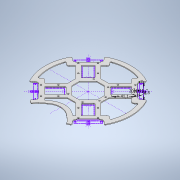
# Autodesk Inventor part: wooden_plate
Saved by Autodesk Inventor 2020 (Build 240168000, 168)
## iProperties
Created: 2023-11-06
Part Number: wooden_plate
Material: Типовые
Document SubType Name: Modeling
Designer: denis
Density: 1 g/cm^3
Appearance: По умолчанию
Author: denis
Autodesk Inventor part; units mm, degrees
ref_plane "YZ Plane" through (0, 0, 0) normal (1, 0, 0) x (0, 1, 0)
ref_plane "XZ Plane" through (0, 0, 0) normal (0, 1, 0) x (-1, 0, 0)
ref_plane "XY Plane" through (0, 0, 0) normal (0, 0, 1) x (1, 0, 0)
sketch "Эскиз1" plane through (0, 0, 0) normal (0, 1, 0) x (-1, 0, 0)
  line L0 (36.7845, -19.8139) -> (61.5324, -44.5618)
  line L1 (36.7845, -5.6718) -> (68.6034, -37.4907)
  line L2 (37.4907, -68.6034) -> (5.6718, -36.7845)
  line L3 (0, 0) -> (60.1181, -60.1181) construction
  line L4 (19.8139, -36.7845) -> (44.5618, -61.5324)
  line L5 (32.2885, -89.3342) -> (30.5289, -89.9833)
  arc A0 (-49.5952, -92.5729) -> (48.7112, -93.0411) centre (0, 0) ccw
  arc A1 (-33.5718, -88.8929) -> (30.5289, -89.9833) centre (0, 0) ccw
  arc A2 (36.7845, -19.8139) -> (33.956, -19.8139) centre (35.3703, -21.2281) ccw
  arc A3 (19.8139, -33.956) -> (19.8139, -36.7845) centre (21.2281, -35.3703) ccw
  line L6 (33.956, -19.8139) -> (19.8139, -33.956)
  arc A4 (48.717, 93.0381) -> (45.4357, 94.6838) centre (0, 0) ccw
  line L7 (0, 0) -> (0, 95.3237) construction
  arc A5 (89.9833, 30.5289) -> (-89.9833, 30.5289) centre (0, 0) ccw construction
  line L8 (0, 0) -> (74.2611, 74.2611) construction
  arc A6 (73.9076, 46.3304) -> (85.2213, 46.3304) centre (79.5644, 51.9873) ccw
  line L9 (85.2213, 46.3304) -> (87.5799, 48.689)
  line L10 (-52.2189, 91.1187) -> (-48.7112, 93.0411) construction
  spline S0 degree 2 poles (-48.6736, 87.5645) (-52.2189, 91.1187) (-48.7112, 93.0411) knots 1 1 1 2 2 2
  line L11 (-48.6736, 87.5645) -> (-52.2189, 91.1187) construction
  arc A7 (-46.3155, 73.8927) -> (-46.3155, 85.2064) centre (-51.9723, 79.5495) ccw
  line L12 (-48.6736, 87.5645) -> (-46.3155, 85.2064)
  arc A8 (-45.4357, 94.6838) -> (-48.7112, 93.0411) centre (0, 0) ccw
  line L13 (-46.3155, 73.8927) -> (-73.8927, 46.3155)
  arc A9 (-85.2064, 46.3155) -> (-73.8927, 46.3155) centre (-79.5495, 51.9723) ccw
  line L14 (-85.2064, 46.3155) -> (-87.5645, 48.6736)
  spline S1 degree 2 poles (-87.5645, 48.6736) (-91.1186, 52.2191) (-92.5729, 49.5952) knots 1 1 1 2 2 2
  line L15 (-87.5645, 48.6736) -> (-91.1186, 52.2191) construction
  line L16 (-91.1186, 52.2191) -> (-92.5729, 49.5952) construction
  arc A10 (44.0429, 95.3397) -> (43.5857, 95.5495) centre (0, 0) ccw construction
  arc A11 (46.3304, 85.2213) -> (46.3304, 73.9076) centre (51.9873, 79.5644) ccw
  line L17 (48.689, 87.5799) -> (46.3304, 85.2213)
  spline S2 degree 2 poles (48.689, 87.5799) (52.2246, 91.1154) (48.717, 93.0381) knots 1 1 1 2 2 2
  line L18 (48.689, 87.5799) -> (52.2246, 91.1154) construction
  line L19 (52.2246, 91.1154) -> (48.717, 93.0381) construction
  line L20 (52.2246, 91.1154) -> (48.689, 87.5799) construction
  line L21 (52.2246, 91.1154) -> (48.689, 87.5799) construction
  line L22 (46.3304, 73.9076) -> (73.9076, 46.3304)
  line L23 (91.1154, 52.2246) -> (87.5799, 48.689) construction
  line L24 (91.1154, 52.2246) -> (92.5699, 49.6008) construction
  spline S3 degree 2 poles (87.5799, 48.689) (91.1154, 52.2246) (92.5699, 49.6008) knots 1 1 1 2 2 2
  line L25 (87.5799, 48.689) -> (91.1154, 52.2246) construction
  arc A12 (-92.5729, 49.5952) -> (-92.5729, -49.5952) centre (0, 0) ccw
  arc A13 (-89.9833, 30.5289) -> (-89.9833, -30.5289) centre (0, 0) ccw
  arc A14 (85.2064, -46.3155) -> (73.9068, -46.3295) centre (79.5636, -51.9864) ccw
  line L26 (85.2064, -46.3155) -> (87.5645, -48.6736)
  arc A15 (92.5729, -49.5952) -> (92.5699, 49.6008) centre (0, 0) ccw
  line L27 (-86.0436, 33.0106) -> (-83.1, 30.067)
  arc A16 (-86.0436, 33.0106) -> (-89.3342, 32.2885) centre (-87.4578, 31.5964) ccw
  line L28 (-89.3342, 32.2885) -> (-89.9833, 30.5289)
  line L29 (91.1154, 52.2246) -> (92.5699, 49.6008) construction
  line L30 (-76.0289, 30.067) -> (-35.2838, 70.8121)
  line L31 (76.0289, 30.067) -> (33.524, 72.5718)
  arc A17 (-48.7112, 93.0411) -> (-92.5729, 49.5952) centre (0, 0) ccw construction
  line L32 (52.2246, 91.1154) -> (48.717, 93.0381) construction
  line L33 (87.5799, 48.689) -> (91.1154, 52.2246) construction
  arc A18 (92.5699, 49.6008) -> (48.717, 93.0381) centre (0, 0) ccw construction
  line L34 (91.1154, 52.2246) -> (52.2246, 91.1154) construction
  line L35 (86.0436, 33.0106) -> (83.1, 30.067)
  arc A19 (89.3342, 32.2885) -> (86.0436, 33.0106) centre (87.4578, 31.5964) ccw
  line L36 (89.3342, 32.2885) -> (89.9833, 30.5289)
  arc A20 (83.7601, -44.8693) -> (89.9833, -30.5289) centre (0, 0) ccw construction
  line L37 (86.0436, -33.0106) -> (83.0991, -30.0661)
  line L38 (89.3342, -32.2885) -> (89.9833, -30.5289)
  arc A21 (86.0436, -33.0106) -> (89.3342, -32.2885) centre (87.4578, -31.5964) ccw
  arc A22 (89.9833, -30.5289) -> (89.9833, 30.5289) centre (0, 0) ccw
  arc A23 (83.0991, -30.0661) -> (76.0281, -30.0661) centre (79.5636, -33.6016) ccw
  arc A24 (30.0661, -76.0281) -> (30.0661, -83.0991) centre (33.6016, -79.5636) ccw
  line L39 (33.0106, -86.0436) -> (30.0661, -83.0991)
  spline S4 degree 2 poles (48.6736, -87.5645) (52.2189, -91.1187) (48.7112, -93.0411) knots 1 1 1 2 2 2
  line L40 (48.6736, -87.5645) -> (52.2189, -91.1187) construction
  line L41 (52.2189, -91.1187) -> (48.7112, -93.0411) construction
  arc A25 (32.2885, -89.3342) -> (33.0106, -86.0436) centre (31.5964, -87.4578) ccw
  line L42 (48.6736, -87.5645) -> (46.3147, -85.2055)
  line L43 (48.6736, -87.5645) -> (46.3147, -85.2055) construction
  arc A26 (46.3295, -73.9068) -> (46.3147, -85.2055) centre (51.9864, -79.5636) ccw
  line L44 (76.0281, -30.0661) -> (30.0661, -76.0281)
  line L45 (46.3295, -73.9068) -> (73.9068, -46.3295)
  line L46 (46.3295, -73.9068) -> (73.9068, -46.3295) construction
  line L47 (73.9068, -46.3295) -> (46.3295, -73.9068) construction
  arc A27 (30.5289, -89.9833) -> (83.7601, -44.8693) centre (0, 0) ccw construction
  line L48 (87.5645, -48.6736) -> (91.1186, -52.2191) construction
  spline S5 degree 2 poles (87.5645, -48.6736) (91.1186, -52.2191) (92.5729, -49.5952) knots 1 1 1 2 2 2
  line L49 (91.1186, -52.2191) -> (92.5729, -49.5952) construction
  arc A28 (48.7112, -93.0411) -> (92.5729, -49.5952) centre (0, 0) ccw construction
  line L50 (0, 51.9187) -> (0, 56.4187) construction
  arc A29 (76.0289, 30.067) -> (83.1, 30.067) centre (79.5644, 33.6025) ccw
  arc A30 (-83.1, 30.067) -> (-76.0289, 30.067) centre (-79.5644, 33.6025) ccw
  line L51 (0, 105) -> (0, 104.941) construction
  arc A31 (-30.0661, -83.0991) -> (-30.0661, -76.0281) centre (-33.6016, -79.5636) ccw
  line L52 (-76.0281, -30.0661) -> (-30.0661, -76.0281)
  arc A32 (-76.0281, -30.0661) -> (-83.0991, -30.0661) centre (-79.5636, -33.6016) ccw
  arc A33 (-33.0106, -86.0436) -> (-32.2885, -89.3342) centre (-31.5964, -87.4578) ccw
  line L53 (-33.0106, -86.0436) -> (-30.0661, -83.0991)
  line L54 (-86.0436, -33.0106) -> (-83.0991, -30.0661)
  arc A34 (-89.3342, -32.2885) -> (-86.0436, -33.0106) centre (-87.4578, -31.5964) ccw
  line L55 (-32.2885, -89.3342) -> (-33.5718, -88.8929)
  line L56 (-89.9833, -30.5289) -> (-89.3342, -32.2885)
  line L57 (-48.6736, -87.5645) -> (-46.3147, -85.2055)
  arc A35 (-46.3147, -85.2055) -> (-46.3295, -73.9068) centre (-51.9864, -79.5636) ccw
  line L58 (-46.3295, -73.9068) -> (-73.9068, -46.3295)
  arc A36 (-73.9068, -46.3295) -> (-85.2064, -46.3155) centre (-79.5636, -51.9864) ccw
  line L59 (-52.2189, -91.1187) -> (-48.7112, -93.0411) construction
  spline S6 degree 2 poles (-48.6736, -87.5645) (-52.2189, -91.1187) (-48.7112, -93.0411) knots 1 1 1 2 2 2
  line L60 (-48.6736, -87.5645) -> (-52.2189, -91.1187) construction
  line L61 (-85.2064, -46.3155) -> (-87.5645, -48.6736)
  line L62 (-87.5645, -48.6736) -> (-91.1186, -52.2191) construction
  spline S7 degree 2 poles (-87.5645, -48.6736) (-91.1186, -52.2191) (-92.5729, -49.5952) knots 1 1 1 2 2 2
  line L63 (-91.1186, -52.2191) -> (-92.5729, -49.5952) construction
  line L64 (95.0211, 0) -> (-95.0211, 0) construction
  line L65 (0, 0) -> (60.1181, 60.1181) construction
  line L66 (33.956, -5.6718) -> (5.6718, -33.956)
  arc A37 (36.7845, -5.6718) -> (33.956, -5.6718) centre (35.3703, -7.086) ccw
  arc A38 (5.6718, -33.956) -> (5.6718, -36.7845) centre (7.086, -35.3703) ccw
  line L67 (-33.956, -19.8139) -> (-19.8139, -33.956)
  arc A39 (-19.8139, -36.7845) -> (-19.8139, -33.956) centre (-21.2281, -35.3703) ccw
  arc A40 (-33.956, -19.8139) -> (-36.7845, -19.8139) centre (-35.3703, -21.2281) ccw
  line L68 (-36.7845, -19.8139) -> (-61.5324, -44.5618)
  line L69 (-36.7845, -5.6718) -> (-68.6034, -37.4907)
  line L70 (0, 0) -> (-60.1181, -60.1181) construction
  line L71 (-37.4907, -68.6034) -> (-5.6718, -36.7845)
  line L72 (-19.8139, -36.7845) -> (-44.5618, -61.5324)
  line L73 (-33.956, -5.6718) -> (-5.6718, -33.956)
  arc A41 (-33.956, -5.6718) -> (-36.7845, -5.6718) centre (-35.3703, -7.086) ccw
  arc A42 (-5.6718, -36.7845) -> (-5.6718, -33.956) centre (-7.086, -35.3703) ccw
  line L74 (33.956, 19.8139) -> (19.8139, 33.956)
  arc A43 (19.8139, 36.7845) -> (19.8139, 33.956) centre (21.2281, 35.3703) ccw
  arc A44 (33.956, 19.8139) -> (36.7845, 19.8139) centre (35.3703, 21.2281) ccw
  line L75 (36.7845, 19.8139) -> (61.5332, 44.5626)
  line L76 (36.7845, 5.6718) -> (68.6043, 37.4916)
  line L77 (0, 0) -> (60.1181, 60.1181) construction
  line L78 (37.4916, 68.6043) -> (5.6718, 36.7845)
  line L79 (19.8139, 36.7845) -> (44.5626, 61.5332)
  line L80 (33.956, 5.6718) -> (5.6718, 33.956)
  arc A45 (5.6718, 36.7845) -> (5.6718, 33.956) centre (7.086, 35.3703) ccw
  arc A46 (-36.7845, 5.6718) -> (-33.956, 5.6718) centre (-35.3703, 7.086) ccw
  line L81 (-33.956, 19.8139) -> (-19.8139, 33.956)
  arc A47 (-19.8139, 33.956) -> (-19.8139, 36.7845) centre (-21.2281, 35.3703) ccw
  line L82 (-36.7845, 5.6718) -> (-68.6043, 37.4916)
  line L83 (-36.7845, 19.8139) -> (-61.5332, 44.5626)
  arc A48 (-36.7845, 19.8139) -> (-33.956, 19.8139) centre (-35.3703, 21.2281) ccw
  line L84 (0, 0) -> (-60.1181, 60.1181) construction
  line L85 (-33.956, 5.6718) -> (-5.6718, 33.956)
  arc A49 (-5.6718, 33.956) -> (-5.6718, 36.7845) centre (-7.086, 35.3703) ccw
  line L86 (-19.8139, 36.7845) -> (-44.5626, 61.5332)
  line L87 (-37.4916, 68.6043) -> (-5.6718, 36.7845)
  arc A50 (33.956, 5.6718) -> (36.7845, 5.6718) centre (35.3703, 7.086) ccw
  line L88 (0, 56.6418) -> (23.7825, 76.5969) construction
  line L89 (52.2091, 91.1) -> (48.6736, 87.5645) construction
  line L90 (52.2091, 91.1) -> (48.6736, 87.5645) construction
  line L91 (48.6736, 87.5645) -> (52.2091, 91.1) construction
  spline S8 degree 2 poles (48.6736, 87.5645) (52.2091, 91.1) (48.7014, 93.0224) knots 1 1 1 2 2 2
  line L92 (52.2091, 91.1) -> (48.7014, 93.0224) construction
  line L93 (52.2091, 91.1) -> (48.7014, 93.0224) construction
  arc A51 (48.7014, 93.0224) -> (44.0271, 95.3237) centre (0, 0) ccw
  arc A52 (44.0271, 95.3237) -> (43.577, 95.5303) centre (0, 0) ccw construction
  line L94 (42.6652, 95.941) -> (43.577, 95.5303) construction
  line L95 (42.6652, 95.941) -> (43.577, 95.5303) construction
  spline S9 degree 2 poles (42.0492, 94.5734) (42.6652, 95.941) (43.577, 95.5303) knots 1 1 1 2 2 2
  line L96 (42.0492, 94.5734) -> (42.6652, 95.941) construction
  line L97 (42.6652, 95.941) -> (42.0492, 94.5734) construction
  spline S10 degree 2 poles (-48.6736, 87.5645) (-52.2091, 91.1) (-48.7014, 93.0224) knots 1 1 1 2 2 2
  line L98 (-48.6736, 87.5645) -> (-52.2091, 91.1) construction
  line L99 (-52.2091, 91.1) -> (-48.7014, 93.0224) construction
  line L100 (0, 56.6418) -> (-35.5516, 86.4744) construction
  line L101 (42.6652, 95.941) -> (-42.6652, 95.941) construction
  ellipse E0 centre (0, 102.7511) end of major axis (44.5159, 105.2445) minor radius 28.887 (35.2734, 86.2384) -> (42.0492, 94.5734) ccw
  line L102 (23.7825, 76.5969) -> (35.2734, 86.2384)
  arc A53 (0, 67.941) -> (23.7825, 76.5969) centre (0, 104.941) ccw
  arc A54 (-23.7825, 76.5969) -> (0, 67.941) centre (0, 104.941) ccw
  line L103 (-23.7825, 76.5969) -> (-35.2734, 86.2384)
  line L104 (-42.6652, 95.941) -> (-42.0492, 94.5734) construction
  arc A55 (-43.577, 95.5303) -> (-48.7014, 93.0224) centre (0, 0) ccw
  line L105 (-42.6652, 95.941) -> (-43.577, 95.5303) construction
  spline S11 degree 2 poles (-42.0492, 94.5734) (-42.6652, 95.941) (-43.577, 95.5303) knots 1 1 1 2 2 2
  line L106 (-42.0492, 94.5734) -> (-42.6652, 95.941) construction
  line L107 (-42.6652, 95.941) -> (-43.577, 95.5303) construction
  line L108 (-42.6652, 95.941) -> (-43.577, 95.5303) construction
  spline S12 degree 2 poles (-42.0492, 94.5734) (-42.6652, 95.941) (-43.577, 95.5303) knots 1 1 1 2 2 2 construction
  line L109 (-42.0492, 94.5734) -> (-42.6652, 95.941) construction
  ellipse E1 centre (0, 102.7511) end of major axis (-44.5159, 105.2445) minor radius 28.887 (-42.0492, 94.5734) -> (-35.2734, 86.2384) ccw
  line L110 (-32.584, 70.9299) -> (-29.9483, 68.7182)
  arc A56 (2.6724, 58.8841) -> (26.0915, 68.7182) centre (-1.9284, 102.6429) ccw
  arc A57 (-29.9483, 68.7182) -> (2.6724, 58.8841) centre (-1.9284, 102.6429) ccw
  line L111 (30.8242, 72.6896) -> (26.0915, 68.7182)
  line L112 (44.0271, 95.3237) -> (43.577, 95.5303)
  arc A58 (33.524, 72.5718) -> (30.8242, 72.6896) centre (32.1098, 71.1576) ccw
  arc A59 (-32.584, 70.9299) -> (-35.2838, 70.8121) centre (-33.8696, 69.3978) ccw
  line L113 (40.3703, 9.2576) -> (40.3703, -9.2576)
  line L114 (35.3703, 5.086) -> (35.3703, -5.086) construction
  line L115 (30.3703, 9.2576) -> (30.3703, -9.2576)
  line L116 (-40.3703, 9.2576) -> (-40.3703, -9.2576)
  line L117 (-30.3703, 9.2576) -> (-30.3703, -9.2576)
  line L118 (-9.2576, -40.3703) -> (9.2576, -40.3703)
  line L119 (-9.2576, -30.3703) -> (9.2576, -30.3703)
  line L120 (-9.2576, 30.3703) -> (9.2576, 30.3703)
  line L121 (-9.2576, 40.3703) -> (9.2576, 40.3703)
  point P0 (35.2199, -88.2529)
  point P1 (35.3703, -4.2576)
  point P2 (4.2576, -35.3703)
  point P3 (0, 66.2701)
  point P4 (88.2529, 35.2199)
  point P5 (-37.2564, 87.4126)
  point P6 (60.119, 60.119)
  point P7 (53.0479, 53.0479)
  point P8 (40.6736, 79.5644)
  point P9 (79.5644, 40.6736)
  point P10 (-83.085, 30.052)
  point P11 (-76.0289, 30.067)
  point P12 (-35.1824, 70.9135)
  point P13 (-53.0479, 53.0479)
  point P14 (35.1824, 70.9135)
  point P15 (76.0289, 30.067)
  point P16 (79.5644, 26.5314)
  point P17 (-44.0429, 95.3397)
  point P18 (83.085, 30.052)
  point P19 (88.2529, 35.2199)
  point P20 (88.2529, -35.2199)
  point P21 (-60.119, 60.119)
  point P22 (79.5644, 26.5314)
  point P23 (73.9066, -74.614)
  point P24 (-4.2576, -35.3703)
  point P25 (-35.3703, -4.2576)
  point P26 (4.2576, 35.3703)
  point P27 (61.5324, 44.5618)
  point P28 (68.6034, 37.4907)
  point P29 (37.4907, 68.6034)
  point P30 (44.5618, 61.5324)
  point P31 (-68.6034, 37.4907)
  point P32 (-61.5324, 44.5618)
  point P33 (-4.2576, 35.3703)
  point P34 (-44.5618, 61.5324)
  point P35 (-37.4907, 68.6034)
  point P36 (74.2462, 74.2462)
  point P37 (40.6586, 79.5495)
  point P38 (92.5543, 49.5852)
  point P39 (0, 105)
  point P40 (-23.542, 76.3968)
  point P41 (-34.9935, 86.0061)
  point P42 (0, 95.941)
  point P43 (-13.2817, 58.6489)
  point P44 (-30.4736, 69.159)
  point P45 (-32.5677, 70.9163)
  point P46 (13.2817, 58.6489)
  point P47 (-23.6028, 54.3247)
  point P48 (-15.6369, 71.4076)
  point P49 (-50.0773, 89.3713)
  point P50 (-48.7112, -93.0411)
  dimension "d84" = 44.5856
  dimension "d0" = 16.3356
  dimension "d1" = 27.5
  dimension "d2" = 8
  dimension "d3" = 5
  dimension "d4" = 5
  dimension "d5" = 3
  dimension "d6" = 4
  dimension "d12" = 5.21
  dimension "d14" = 10
  dimension "d15" = 10
  dimension "d16" = 10
  dimension "d22" = 5
  dimension "d23" = 2
  dimension "d24" = 10
  dimension "d25" = 10
  dimension "d26" = 10
  dimension "d27" = 5
  dimension "d28" = 2
  dimension "d29" = 5
  dimension "d30" = 5
  dimension "d31" = 2
  dimension "d41" = 36.9988
  dimension "d43" = 10
  dimension "d44" = 10
  dimension "d45" = 12
  dimension "d46" = 12
  dimension "d47" = 2
  dimension "d56" = 5
  dimension "d57" = 5
  dimension "d58" = 0.059
  dimension "d68" = 20
  dimension "d70" = 20
  dimension "d71" = 66.9988
  dimension "d72" = 10
  dimension "d74" = 100
  dimension "d75" = 28
  dimension "d76" = 15
  dimension "d78" = 5
  dimension "d79" = 1
  dimension "d80" = 1.5
  dimension "d81" = 1.5
  dimension "d82" = 1
  dimension "d83" = 4
  dimension "d85" = 10
  dimension "d87" = 2
  dimension "d89" = 5
  constraints: 190 end point, 152 point on circle, 103 symmetric about line, 59 centre point, 56 point on line, 30 tangent, 25 coincident, 13 parallel, 9 collinear, 5 equal radius, 5 perpendicular, 3 midpoint, 3 vertical, 101 other
  measures "d0" distance of L34.start point (79.564, 40.674)
  measures "d1" distance of point (40.674, 79.564) point (60.119, 60.119)
  measures "d2" radius of A11
  measures "d3" distance of L32.start L20.end
  measures "d4" distance of L9.end L34.start
  measures "d5" distance of L34.start L24.end
  measures "d6" distance of L32.start L19.end
  measures "d12" distance of A10.start L19.end
  measures "d14" radial gap between concentric circles of A15 A5
  measures "d16" distance between parallel lines of L9 L35
  measures "d22" distance of point (88.253, 35.22) L36.end
  measures "d23" radius of A19
  measures "d24" distance between parallel lines of L37 L26
  measures "d25" distance between parallel lines of L42 L39
  measures "d26" distance between parallel lines of L44 L45
  measures "d27" distance of point (88.253, -35.22) L38.end
  measures "d28" radius of A21
  measures "d29" radius of A23
  measures "d30" distance of point (35.22, -88.253) L5.end
  measures "d31" radius of A25
  measures "d41" distance between parallel lines of L6 L44
  measures "d43" distance between parallel lines of L1 L0
  measures "d44" distance between parallel lines of L2 L4
  measures "d45" distance between parallel lines of L3 L4
  measures "d46" distance between parallel lines of L0 L3
  measures "d47" radius of A2
  measures "d56" radius of A29
  measures "d57" radius of A30
  measures "d58" distance of L51.start L51.end
  measures "d68" distance from line of L45 point (73.907, -74.614)
  measures "d70" distance from line of L8.end L22
  measures "d71" distance from line of point (73.907, -74.614) L6
  measures "d72" distance between parallel lines of L6 L66
  measures "d74" angle of L100 L88
  measures "d75" distance from line of L101 A53.start
  measures "d76" distance of L88.end L102.end
  measures "d78" distance of L89.start L89.end
  measures "d79" distance of L97.start L95.end
  measures "d80" distance of L97.start L97.end
  measures "d81" distance of L104.start L104.end
  measures "d82" distance of L104.start L108.end
  measures "d83" distance of L89.start L92.end
  measures "d85" distance between parallel lines of L100 L110
  measures "d87" radius of A58
  measures "d89" distance between parallel lines of L113 L114
sketch "Эскиз2" plane through (0, 0, 0) normal (0, 1, 0) x (-1, 0, 0)
  point P0 (0, 0)
extrude "Выдавливание1" add sketch "Эскиз1" along normal blind 2 contours A2 L6 A3 L4 L44 L2 A38 L66 A37 L1 L0 | L1 A37 L66 L115 L80 A50 L76 L113 | L76 A50 L80 A45 L78 L31 L79 A43 L74 A44 L75 | L118 L71 A42 L73 L119 L66 A38 L2 | L71 L52 L72 A39 L67 A40 L68 L69 A41 L73 A42 | L120 L85 A49 L87 L121 L78 A45 L80 | L73 A41 L69 L116 L82 A46 L85 L117 | L85 A46 L82 L30 L83 A48 L81 A47 L86 L87 A49 | S6 L57 A35 L58 A36 L61 S7 A12 S1 L14 A9 L13 A7 L12 S10 A55 S11 E1 L103 A54 A53 L102 E0 S9 L112 A51 S8 L17 A11 L22 A6 L9 S3 A15 S5 L26 A14 L45 A26 L42 S4 A0
sketch "Эскиз3" plane through (0, 2, 0) normal (0, 1, 0) x (1, 0, 0)
  line L0 (46.3155, -73.8927) -> (73.8927, -46.3155) projected
  arc A0 (85.2064, -46.3155) -> (73.8927, -46.3155) centre (79.5495, -51.9723) ccw projected
  line L1 (85.2064, -46.3155) -> (87.5645, -48.6736) projected
  arc A1 (92.5729, -49.5952) -> (92.5729, 49.5952) centre (0, 0) ccw projected
  line L2 (87.5645, 48.6736) -> (85.2064, 46.3155) projected
  arc A2 (73.9068, 46.3295) -> (85.2064, 46.3155) centre (79.5636, 51.9864) ccw projected
  line L3 (73.9068, 46.3295) -> (46.3295, 73.9068) projected
  arc A3 (46.3147, 85.2055) -> (46.3295, 73.9068) centre (51.9864, 79.5636) ccw projected
  line L4 (46.3147, 85.2055) -> (48.6736, 87.5645) projected
  arc A4 (48.7112, 93.0411) -> (-48.7112, 93.0411) centre (0, 0) ccw projected
  line L5 (-48.6736, 87.5645) -> (-46.3147, 85.2055) projected
  arc A5 (-46.3295, 73.9068) -> (-46.3147, 85.2055) centre (-51.9864, 79.5636) ccw projected
  line L6 (-46.3295, 73.9068) -> (-73.9068, 46.3295) projected
  arc A6 (-85.2064, 46.3155) -> (-73.9068, 46.3295) centre (-79.5636, 51.9864) ccw projected
  line L7 (-85.2064, 46.3155) -> (-87.5645, 48.6736) projected
  arc A7 (-92.5729, 49.5952) -> (-92.5699, -49.6008) centre (0, 0) ccw projected
  line L8 (-87.5799, -48.689) -> (-85.2213, -46.3304) projected
  arc A8 (-73.9076, -46.3304) -> (-85.2213, -46.3304) centre (-79.5644, -51.9873) ccw projected
  line L9 (-73.9076, -46.3304) -> (-46.3304, -73.9076) projected
  arc A9 (-46.3304, -85.2213) -> (-46.3304, -73.9076) centre (-51.9873, -79.5644) ccw projected
  line L10 (-46.3304, -85.2213) -> (-48.6736, -87.5645) projected
  arc A10 (-48.7014, -93.0224) -> (-44.0271, -95.3237) centre (0, 0) ccw projected
  line L11 (-44.0271, -95.3237) -> (-43.577, -95.5303) projected
  ellipse E0 centre (0, -102.7511) end of major axis (44.5159, -100.2577) minor radius 28.887 (-35.2734, -86.2384) -> (-42.0492, -94.5734) ccw projected
  line L12 (-35.2734, -86.2384) -> (-23.7825, -76.5969) projected
  arc A11 (23.7825, -76.5969) -> (-23.7825, -76.5969) centre (0, -104.941) ccw projected
  line L13 (23.7825, -76.5969) -> (35.2734, -86.2384) projected
  ellipse E1 centre (0, -102.7511) end of major axis (-44.5159, -100.2577) minor radius 28.887 (42.0492, -94.5734) -> (35.2734, -86.2384) ccw projected
  arc A12 (43.577, -95.5303) -> (48.7014, -93.0224) centre (0, 0) ccw projected
  line L14 (48.6736, -87.5645) -> (46.3155, -85.2064) projected
  arc A13 (46.3155, -73.8927) -> (46.3155, -85.2064) centre (51.9723, -79.5495) ccw projected
  arc A14 (83.1, -30.067) -> (76.0289, -30.067) centre (79.5644, -33.6025) ccw projected
  line L15 (76.0289, -30.067) -> (68.6043, -37.4916) projected
  line L16 (68.6043, -37.4916) -> (40.3703, -9.2576) projected
  line L17 (40.3703, -9.2576) -> (40.3703, 9.2576) projected
  line L18 (40.3703, 9.2576) -> (68.6034, 37.4907) projected
  line L19 (68.6034, 37.4907) -> (76.0281, 30.0661) projected
  arc A15 (76.0281, 30.0661) -> (83.0991, 30.0661) centre (79.5636, 33.6016) ccw projected
  line L20 (83.0991, 30.0661) -> (86.0436, 33.0106) projected
  arc A16 (89.3342, 32.2885) -> (86.0436, 33.0106) centre (87.4578, 31.5964) ccw projected
  line L21 (89.3342, 32.2885) -> (89.9833, 30.5289) projected
  arc A17 (89.9833, -30.5289) -> (89.9833, 30.5289) centre (0, 0) ccw projected
  line L22 (89.9833, -30.5289) -> (89.3342, -32.2885) projected
  arc A18 (86.0436, -33.0106) -> (89.3342, -32.2885) centre (87.4578, -31.5964) ccw projected
  line L23 (86.0436, -33.0106) -> (83.1, -30.067) projected
  line L24 (-30.3703, 9.2576) -> (-9.2576, 30.3703) projected
  line L25 (-9.2576, 30.3703) -> (9.2576, 30.3703) projected
  line L26 (9.2576, 30.3703) -> (30.3703, 9.2576) projected
  line L27 (30.3703, 9.2576) -> (30.3703, -9.2576) projected
  line L28 (30.3703, -9.2576) -> (9.2576, -30.3703) projected
  line L29 (9.2576, -30.3703) -> (-9.2576, -30.3703) projected
  line L30 (-9.2576, -30.3703) -> (-30.3703, -9.2576) projected
  line L31 (-30.3703, -9.2576) -> (-30.3703, 9.2576) projected
  line L32 (-68.6043, -37.4916) -> (-76.0289, -30.067) projected
  arc A19 (-76.0289, -30.067) -> (-83.1, -30.067) centre (-79.5644, -33.6025) ccw projected
  line L33 (-83.1, -30.067) -> (-86.0436, -33.0106) projected
  arc A20 (-89.3342, -32.2885) -> (-86.0436, -33.0106) centre (-87.4578, -31.5964) ccw projected
  line L34 (-89.3342, -32.2885) -> (-89.9833, -30.5289) projected
  arc A21 (-89.9833, 30.5289) -> (-89.9833, -30.5289) centre (0, 0) ccw projected
  line L35 (-89.9833, 30.5289) -> (-89.3342, 32.2885) projected
  arc A22 (-86.0436, 33.0106) -> (-89.3342, 32.2885) centre (-87.4578, 31.5964) ccw projected
  line L36 (-86.0436, 33.0106) -> (-83.0991, 30.0661) projected
  arc A23 (-83.0991, 30.0661) -> (-76.0281, 30.0661) centre (-79.5636, 33.6016) ccw projected
  line L37 (-76.0281, 30.0661) -> (-68.6034, 37.4907) projected
  line L38 (-68.6034, 37.4907) -> (-40.3703, 9.2576) projected
  line L39 (-40.3703, 9.2576) -> (-40.3703, -9.2576) projected
  line L40 (-40.3703, -9.2576) -> (-68.6043, -37.4916) projected
  arc A24 (33.5718, 88.8929) -> (-30.5289, 89.9833) centre (0, 0) ccw projected
  line L41 (33.5718, 88.8929) -> (32.2885, 89.3342) projected
  arc A25 (33.0106, 86.0436) -> (32.2885, 89.3342) centre (31.5964, 87.4578) ccw projected
  line L42 (33.0106, 86.0436) -> (30.0661, 83.0991) projected
  arc A26 (30.0661, 83.0991) -> (30.0661, 76.0281) centre (33.6016, 79.5636) ccw projected
  line L43 (30.0661, 76.0281) -> (37.4907, 68.6034) projected
  line L44 (37.4907, 68.6034) -> (9.2576, 40.3703) projected
  line L45 (9.2576, 40.3703) -> (-9.2576, 40.3703) projected
  line L46 (-9.2576, 40.3703) -> (-37.4907, 68.6034) projected
  line L47 (-37.4907, 68.6034) -> (-30.0661, 76.0281) projected
  arc A27 (-30.0661, 76.0281) -> (-30.0661, 83.0991) centre (-33.6016, 79.5636) ccw projected
  line L48 (-30.0661, 83.0991) -> (-33.0106, 86.0436) projected
  arc A28 (-32.2885, 89.3342) -> (-33.0106, 86.0436) centre (-31.5964, 87.4578) ccw projected
  line L49 (-32.2885, 89.3342) -> (-30.5289, 89.9833) projected
  line L50 (-61.5332, -44.5626) -> (-36.7845, -19.8139) projected
  arc A29 (-33.956, -19.8139) -> (-36.7845, -19.8139) centre (-35.3703, -21.2281) ccw projected
  line L51 (-33.956, -19.8139) -> (-19.8139, -33.956) projected
  arc A30 (-19.8139, -36.7845) -> (-19.8139, -33.956) centre (-21.2281, -35.3703) ccw projected
  line L52 (-19.8139, -36.7845) -> (-44.5626, -61.5332) projected
  line L53 (-44.5626, -61.5332) -> (-61.5332, -44.5626) projected
  arc A31 (-36.7845, 19.8139) -> (-33.956, 19.8139) centre (-35.3703, 21.2281) ccw projected
  line L54 (-36.7845, 19.8139) -> (-61.5324, 44.5618) projected
  line L55 (-61.5324, 44.5618) -> (-44.5618, 61.5324) projected
  line L56 (-44.5618, 61.5324) -> (-19.8139, 36.7845) projected
  arc A32 (-19.8139, 33.956) -> (-19.8139, 36.7845) centre (-21.2281, 35.3703) ccw projected
  line L57 (-19.8139, 33.956) -> (-33.956, 19.8139) projected
  line L58 (61.5324, 44.5618) -> (36.7845, 19.8139) projected
  arc A33 (33.956, 19.8139) -> (36.7845, 19.8139) centre (35.3703, 21.2281) ccw projected
  line L59 (33.956, 19.8139) -> (19.8139, 33.956) projected
  arc A34 (19.8139, 36.7845) -> (19.8139, 33.956) centre (21.2281, 35.3703) ccw projected
  line L60 (19.8139, 36.7845) -> (44.5618, 61.5324) projected
  line L61 (44.5618, 61.5324) -> (61.5324, 44.5618) projected
  arc A35 (36.7845, -19.8139) -> (33.956, -19.8139) centre (35.3703, -21.2281) ccw projected
  line L62 (36.7845, -19.8139) -> (61.5332, -44.5626) projected
  line L63 (61.5332, -44.5626) -> (44.5626, -61.5332) projected
  line L64 (44.5626, -61.5332) -> (19.8139, -36.7845) projected
  arc A36 (19.8139, -33.956) -> (19.8139, -36.7845) centre (21.2281, -35.3703) ccw projected
  line L65 (19.8139, -33.956) -> (33.956, -19.8139) projected
  line L66 (9.2576, -40.3703) -> (37.4916, -68.6043) projected
  line L67 (37.4916, -68.6043) -> (35.2838, -70.8121) projected
  arc A37 (32.584, -70.9299) -> (35.2838, -70.8121) centre (33.8696, -69.3978) ccw projected
  line L68 (32.584, -70.9299) -> (29.9483, -68.7182) projected
  arc A38 (29.9483, -68.7182) -> (-26.0915, -68.7182) centre (1.9284, -102.6429) ccw projected
  line L69 (-26.0915, -68.7182) -> (-30.8242, -72.6896) projected
  arc A39 (-33.524, -72.5718) -> (-30.8242, -72.6896) centre (-32.1098, -71.1576) ccw projected
  line L70 (-33.524, -72.5718) -> (-37.4916, -68.6043) projected
  line L71 (-37.4916, -68.6043) -> (-9.2576, -40.3703) projected
  line L72 (-9.2576, -40.3703) -> (9.2576, -40.3703) projected
  line L73 (17.5, -31.25) -> (-17.5, -31.25) construction
  line L74 (-17.5, -31.25) -> (-17.5, 31.25) construction
  line L75 (-17.5, 31.25) -> (17.5, 31.25) construction
  line L76 (17.5, 31.25) -> (17.5, -31.25) construction
  circle A40 centre (-17.5, -31.25) radius 1.75
  circle A41 centre (17.5, -31.25) radius 1.75
  circle A42 centre (-17.5, 31.25) radius 1.75
  circle A43 centre (17.5, 31.25) radius 1.75
  line L77 (0, -181.7301) -> (0, 190.7859) construction
  line L78 (191.5563, 0) -> (-204.2421, 0) construction
  line L79 (0, -31.25) -> (0, 31.25) construction
  line L80 (17.5, 0) -> (-17.5, 0) construction
  circle A44 centre (69.65, -45.6084) radius 1.75
  circle A45 centre (45.6084, -69.65) radius 1.75
  line L81 (69.65, -45.6084) -> (45.6084, -69.65) construction
  line L82 (61.5332, -44.5626) -> (44.5626, -61.5332) construction
  line L83 (0, 0) -> (87.7902, -87.7902) construction
  circle A46 centre (-69.65, -45.6084) radius 1.75
  circle A47 centre (-45.6084, -69.65) radius 1.75
  circle A48 centre (69.65, 45.6084) radius 1.75
  circle A49 centre (45.6084, 69.65) radius 1.75
  circle A50 centre (-45.6084, 69.65) radius 1.75
  circle A51 centre (-69.65, 45.6084) radius 1.75
  circle A52 centre (48.4368, -24.3952) radius 1.75
  circle A53 centre (24.3952, -48.4368) radius 1.75
  line L84 (48.4368, -24.3952) -> (24.3952, -48.4368) construction
  circle A54 centre (-24.3952, -48.4368) radius 1.75
  circle A55 centre (-48.4368, -24.3952) radius 1.75
  circle A56 centre (24.3952, 48.4368) radius 1.75
  circle A57 centre (48.4368, 24.3952) radius 1.75
  circle A58 centre (-24.3952, 48.4368) radius 1.75
  circle A59 centre (-48.4368, 24.3952) radius 1.75
  line L85 (146.7, -29.0626) -> (121.7, -29.0626) construction
  line L86 (121.7, -29.0626) -> (121.7, -9.0626) construction
  line L87 (121.7, -9.0626) -> (146.7, -9.0626) construction
  line L88 (146.7, -9.0626) -> (146.7, -29.0626) construction
  circle A60 centre (124.2, -26.5626) radius 1.75
  line L89 (121.7, -19.0626) -> (146.7, -19.0626) construction
  circle A61 centre (124.2, -11.5626) radius 1.75
  line L90 (124.2, -26.5626) -> (124.2, -11.5626) construction
  line L91 (13.5, 54.0187) -> (-13.5, 54.0187) construction
  line L92 (-13.5, 54.0187) -> (-13.5, 81.0187) construction
  line L93 (-13.5, 81.0187) -> (13.5, 81.0187) construction
  line L94 (13.5, 81.0187) -> (13.5, 54.0187) construction
  circle A62 centre (13.5, 54.0187) radius 1.75
  circle A63 centre (-13.5, 54.0187) radius 1.75
  circle A64 centre (13.5, 81.0187) radius 1.75
  circle A65 centre (-13.5, 81.0187) radius 1.75
  line L95 (0, 54.0187) -> (0, 81.0187) construction
  circle A66 centre (35.3703, -7.65) radius 1.75
  circle A67 centre (35.3703, 7.65) radius 1.75
  line L96 (35.3703, -7.65) -> (35.3703, 7.65) construction
  line L97 (32.6703, -10.6) -> (32.6703, 10.6) construction
  line L98 (32.6703, 10.6) -> (47.1703, 10.6) construction
  line L99 (47.1703, 10.6) -> (47.1703, -10.6) construction
  line L100 (47.1703, -10.6) -> (32.6703, -10.6) construction
  line L101 (32.6703, 0) -> (47.1703, 0) construction
  line L102 (40.3703, -9.2576) -> (40.3703, 9.2576) construction
  line L103 (20.5, -34.5) -> (-20.5, -34.5) construction
  line L104 (-20.5, -34.5) -> (-20.5, 34.5) construction
  line L105 (-20.5, 34.5) -> (20.5, 34.5) construction
  line L106 (20.5, 34.5) -> (20.5, -34.5) construction
  point P0 (50.0773, -89.3713)
  point P1 (57.6292, -57.6292)
  point P2 (36.416, -36.416)
  point P3 (35.3703, 0)
  point P4 (0, -34.5)
  point P5 (0, 34.5)
  point P6 (-20.5, 0)
  point P7 (20.5, 0)
  dimension "d92" = 35
  dimension "d93" = 62.5
  dimension "d94" = 3.5
  dimension "d95" = 3.5
  dimension "d96" = 3.5
  dimension "d97" = 3.5
  dimension "d108" = 3.5
  dimension "d109" = 3.5
  dimension "d110" = 34
  dimension "d112" = 3.5
  dimension "d113" = 3.5
  dimension "d114" = 3.5
  dimension "d115" = 34
  dimension "d116" = 30
  dimension "d117" = 25
  dimension "d118" = 20
  dimension "d119" = 3.5
  dimension "d122" = 15
  dimension "d123" = 2.5
  dimension "d124" = 27
  dimension "d125" = 27
  dimension "d126" = 3.5
  dimension "d127" = 3.5
  dimension "d128" = 3.5
  dimension "d129" = 3.5
  dimension "d130" = 3.5
  dimension "d131" = 3.5
  dimension "d132" = 15.3
  dimension "d133" = 21.2
  dimension "d135" = 2.7
  dimension "d136" = 14.5
  dimension "d137" = 41
  dimension "d138" = 69
  dimension "d139" = 5
  dimension "d140" = 45
  constraints: 64 end point, 28 centre point, 17 midpoint, 13 parallel, 13 symmetric about line, 8 coincident, 6 horizontal, 6 perpendicular, 5 point on line, 4 collinear, 3 vertical, 26 other
  measures "d92" distance of L73.start L73.end
  measures "d93" distance of L75.end L73.start
  measures "d94" diameter of A40
  measures "d95" diameter of A41
  measures "d96" diameter of A42
  measures "d97" diameter of A43
  measures "d108" diameter of A44
  measures "d109" diameter of A45
  measures "d110" distance of L81.start L81.end
  measures "d112" distance between parallel lines of L0 L81
  measures "d113" diameter of A52
  measures "d114" diameter of A53
  measures "d115" distance of L84.start L84.end
  measures "d116" distance between parallel lines of L84 L81
  measures "d117" distance of L86.end L87.end
  measures "d118" distance of L85.end L86.end
  measures "d119" diameter of A60
  measures "d122" distance of L90.end L90.start
  measures "d123" distance between parallel lines of L86 L90
  measures "d124" distance of L92.end L93.end
  measures "d125" distance of L91.end L92.end
  measures "d126" diameter of A62
  measures "d127" diameter of A63
  measures "d128" diameter of A64
  measures "d129" diameter of A65
  measures "d130" diameter of A66
  measures "d131" diameter of A67
  measures "d132" distance of L96.start L96.end
  measures "d133" distance of L98.end L99.end
  measures "d135" distance between parallel lines of L97 L96
  measures "d136" distance of L99.end L97.start
  measures "d137" distance of L104.end L105.end
  measures "d138" distance of L103.end L104.end
  measures "d139" distance between parallel lines of L27 L96
  measures "d140" angle of L79 L83
sketch "моторы" plane through (0, 0, 0) normal (0, 1, 0) x (-1, 0, 0)
  arc A0 (-51.9723, -82.3779) -> (-47.0226, -77.4282) centre (-49.4975, -79.9031) ccw
  line L0 (-44.5477, -79.9031) -> (-49.4975, -84.8528) construction
  line L1 (0, 0) -> (-79.4987, -79.4987) construction
  line L2 (-21.7082, -36.1332) -> (-50.7703, -65.1952) construction
  line L3 (-50.7703, -65.1952) -> (-65.1952, -50.7703) construction
  line L4 (-65.1952, -50.7703) -> (-36.1332, -21.7082) construction
  line L5 (-36.1332, -21.7082) -> (-21.7082, -36.1332) construction
  line L6 (-28.9207, -28.9207) -> (-57.9828, -57.9828) construction
  line L7 (-69.8885, -50.3196) -> (-42.3114, -77.8968) construction
  line L8 (-57.6292, -62.579) -> (-55.5079, -60.4576) construction
  line L9 (-61.3415, -58.8666) -> (-58.8666, -61.3415) construction
  line L10 (-57.9828, -57.9828) -> (-60.1041, -60.1041) construction
  line L11 (-69.4732, -71.9481) -> (-71.9481, -69.4732) construction
  line L12 (-67.1751, -67.1751) -> (-62.2254, -62.2254) construction
  line L13 (-62.579, -57.6292) -> (-57.6292, -62.579) construction
  line L14 (-55.5079, -60.4576) -> (-60.4576, -55.5079) construction
  line L15 (-58.8666, -61.3415) -> (-69.4732, -71.9481) construction
  line L16 (-60.1041, -60.1041) -> (-70.7107, -70.7107) construction
  line L17 (-49.4975, -84.8528) -> (-84.8528, -49.4975) construction
  line L18 (-79.9031, -44.5477) -> (-44.5477, -79.9031) construction
  line L19 (-71.9481, -69.4732) -> (-61.3415, -58.8666) construction
  line L20 (-60.4576, -55.5079) -> (-62.579, -57.6292) construction
  arc A1 (-77.4282, -47.0226) -> (-82.3779, -51.9723) centre (-79.9031, -49.4975) ccw
  line L21 (-84.8528, -49.4975) -> (-79.9031, -44.5477) construction
  line L22 (0, 0) -> (74.2462, 74.2462) construction
  line L23 (-46.3155, -73.8927) -> (-73.8927, -46.3155)
  line L24 (0, 0) -> (0, 95.3237) construction
  arc A2 (82.3779, -51.9723) -> (77.4282, -47.0226) centre (79.9031, -49.4975) ccw
  line L25 (84.8528, -49.4975) -> (79.9031, -44.5477) construction
  line L26 (58.8666, -61.3415) -> (69.4732, -71.9481) construction
  line L27 (67.1751, -67.1751) -> (62.2254, -62.2254) construction
  line L28 (0, 0) -> (79.4987, -79.4987) construction
  line L29 (21.7082, -36.1332) -> (50.7703, -65.1952) construction
  line L30 (65.1952, -50.7703) -> (36.1332, -21.7082) construction
  line L31 (28.9207, -28.9207) -> (57.9828, -57.9828) construction
  line L32 (60.4576, -55.5079) -> (62.579, -57.6292) construction
  line L33 (61.3415, -58.8666) -> (58.8666, -61.3415) construction
  line L34 (57.9828, -57.9828) -> (60.1041, -60.1041) construction
  line L35 (69.4732, -71.9481) -> (71.9481, -69.4732) construction
  line L36 (62.579, -57.6292) -> (57.6292, -62.579) construction
  line L37 (55.5079, -60.4576) -> (60.4576, -55.5079) construction
  line L38 (71.9481, -69.4732) -> (61.3415, -58.8666) construction
  line L39 (57.6292, -62.579) -> (55.5079, -60.4576) construction
  line L40 (60.1041, -60.1041) -> (70.7107, -70.7107) construction
  line L41 (50.7703, -65.1952) -> (65.1952, -50.7703) construction
  line L42 (49.4975, -84.8528) -> (84.8528, -49.4975) construction
  line L43 (79.9031, -44.5477) -> (44.5477, -79.9031) construction
  line L44 (46.3155, -73.8927) -> (73.8927, -46.3155)
  line L45 (69.8885, -50.3196) -> (42.3114, -77.8968) construction
  arc A3 (47.0226, -77.4282) -> (51.9723, -82.3779) centre (49.4975, -79.9031) ccw
  line L46 (44.5477, -79.9031) -> (49.4975, -84.8528) construction
  line L47 (36.1332, -21.7082) -> (21.7082, -36.1332) construction
  line L48 (98, 0) -> (-98, 0) construction
  line L49 (36.1332, 21.7082) -> (21.7082, 36.1332) construction
  line L50 (21.7082, 36.1332) -> (50.7703, 65.1952) construction
  line L51 (0, 0) -> (79.4987, 79.4987) construction
  line L52 (28.9207, 28.9207) -> (57.9828, 57.9828) construction
  line L53 (65.1952, 50.7703) -> (36.1332, 21.7082) construction
  line L54 (60.4576, 55.5079) -> (62.579, 57.6292) construction
  line L55 (-36.1332, 21.7082) -> (-21.7082, 36.1332) construction
  line L56 (-28.9207, 28.9207) -> (-57.9828, 57.9828) construction
  line L57 (-21.7082, 36.1332) -> (-50.7703, 65.1952) construction
  line L58 (0, 0) -> (-79.4987, 79.4987) construction
  line L59 (-50.7703, 65.1952) -> (-65.1952, 50.7703) construction
  line L60 (-69.8885, 50.3196) -> (-42.3114, 77.8968) construction
  line L61 (-65.1952, 50.7703) -> (-36.1332, 21.7082) construction
  line L62 (-57.6292, 62.579) -> (-55.5079, 60.4576) construction
  line L63 (-57.9828, 57.9828) -> (-60.1041, 60.1041) construction
  line L64 (-55.5079, 60.4576) -> (-60.4576, 55.5079) construction
  line L65 (-61.3415, 58.8666) -> (-58.8666, 61.3415) construction
  line L66 (-62.579, 57.6292) -> (-57.6292, 62.579) construction
  line L67 (-67.1751, 67.1751) -> (-62.2254, 62.2254) construction
  line L68 (-58.8666, 61.3415) -> (-69.4732, 71.9481) construction
  line L69 (-60.1041, 60.1041) -> (-70.7107, 70.7107) construction
  line L70 (-69.4732, 71.9481) -> (-71.9481, 69.4732) construction
  arc A4 (51.9723, 82.3779) -> (47.0226, 77.4282) centre (49.4975, 79.9031) ccw
  line L71 (44.5477, 79.9031) -> (49.4975, 84.8528) construction
  line L72 (57.6292, 62.579) -> (55.5079, 60.4576) construction
  line L73 (57.9828, 57.9828) -> (60.1041, 60.1041) construction
  line L74 (69.4732, 71.9481) -> (71.9481, 69.4732) construction
  line L75 (62.579, 57.6292) -> (57.6292, 62.579) construction
  line L76 (55.5079, 60.4576) -> (60.4576, 55.5079) construction
  line L77 (58.8666, 61.3415) -> (69.4732, 71.9481) construction
  line L78 (50.7703, 65.1952) -> (65.1952, 50.7703) construction
  line L79 (69.8885, 50.3196) -> (42.3114, 77.8968) construction
  line L80 (46.3155, 73.8927) -> (73.8927, 46.3155)
  line L81 (79.9031, 44.5477) -> (44.5477, 79.9031) construction
  line L82 (49.4975, 84.8528) -> (84.8528, 49.4975) construction
  arc A5 (77.4282, 47.0226) -> (82.3779, 51.9723) centre (79.9031, 49.4975) ccw
  line L83 (84.8528, 49.4975) -> (79.9031, 44.5477) construction
  line L84 (61.3415, 58.8666) -> (58.8666, 61.3415) construction
  line L85 (71.9481, 69.4732) -> (61.3415, 58.8666) construction
  line L86 (67.1751, 67.1751) -> (62.2254, 62.2254) construction
  line L87 (60.1041, 60.1041) -> (70.7107, 70.7107) construction
  arc A6 (-47.0226, 77.4282) -> (-51.9723, 82.3779) centre (-49.4975, 79.9031) ccw
  line L88 (-44.5477, 79.9031) -> (-49.4975, 84.8528) construction
  line L89 (-84.8528, 49.4975) -> (-79.9031, 44.5477) construction
  arc A7 (-82.3779, 51.9723) -> (-77.4282, 47.0226) centre (-79.9031, 49.4975) ccw
  line L90 (-71.9481, 69.4732) -> (-61.3415, 58.8666) construction
  line L91 (-46.3155, 73.8927) -> (-73.8927, 46.3155)
  line L92 (-79.9031, 44.5477) -> (-44.5477, 79.9031) construction
  line L93 (-49.4975, 84.8528) -> (-84.8528, 49.4975) construction
  line L94 (-60.4576, 55.5079) -> (-62.579, 57.6292) construction
  point P0 (-56.0999, -64.1082)
  point P1 (56.0999, -64.1082)
  point P2 (56.0999, 64.1082)
  point P3 (-56.0999, 64.1082)
  dimension "d98" = 20.4
  dimension "d99" = 3
  dimension "d100" = 3
  dimension "d101" = 7
  dimension "d102" = 15
  dimension "d103" = 3.5
  dimension "d104" = 7
  dimension "d105" = 50
  dimension "d106" = 3
  dimension "d107" = 41.1
  constraints: 190 end point, 111 symmetric about line, 16 point on circle, 9 midpoint, 8 centre point, 8 collinear, 8 parallel, 8 point on line, 4 perpendicular, 3 tangent, 7 other
  measures "d98" distance of L2.end L3.end
  measures "d99" distance from line of L3 point (-56.1, -64.108)
  measures "d100" distance of L13.end L14.start
  measures "d101" distance of L20.start L14.start
  measures "d102" distance of L15.start L11.start
  measures "d103" distance of L11.start L11.end
  measures "d104" distance of L18.end L17.start
  measures "d105" distance of L17.start L17.end
  measures "d106" distance between parallel lines of L13 L18
  measures "d107" distance of L3.end L4.end
extrude "Выдавливание2" cut sketch "Эскиз3" against normal blind 5 contours A40 | A41 | A42 | A43 | A44 | A45 | A46 | A47 | A48 | A49 | A50 | A51 | A52 | A53 | A54 | A55 | A56 | A57 | A58 | A59 | A66 | A67
